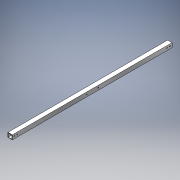
# Autodesk Inventor part: 上昇機構_角柱3
Saved by Autodesk Inventor 2019.4 (Build 234330000, 330)
## iProperties
Created: 2021-12-04
Part Number: 上昇機構_角柱3
Material: アルミニウム 6061
Document SubType Name: Modeling
Designer: 堀川皓史
Density: 2.7 g/cm^3
Appearance: アルミニウム - フラット
Mass: 119.894 g
Surface Area: 595.499 cm^2
Volume: 44.4052 cm^3
Author: 堀川皓史
Autodesk Inventor part; units mm, degrees
ref_plane "YZ Plane" through (0, 0, 0) normal (1, 0, 0) x (0, 1, 0)
ref_plane "XZ Plane" through (0, 0, 0) normal (0, 1, 0) x (-1, 0, 0)
ref_plane "XY Plane" through (0, 0, 0) normal (0, 0, 1) x (1, 0, 0)
sketch "スケッチ1" plane through (0, 0, 0) normal (0, 0, 1) x (1, 0, 0)
  line L0 (7.5, 7.5) -> (-7.5, 7.5)
  line L1 (-7.5, 7.5) -> (-7.5, -7.5)
  line L2 (-7.5, -7.5) -> (7.5, -7.5)
  line L3 (7.5, -7.5) -> (7.5, 7.5)
  line L4 (7.5, 7.5) -> (-7.5, -7.5) construction
  line L5 (-7.5, 7.5) -> (7.5, -7.5) construction
  line L6 (-6, 6) -> (6, 6)
  line L7 (6, 6) -> (6, -6)
  line L8 (6, -6) -> (-6, -6)
  line L9 (-6, -6) -> (-6, 6)
  point P0 (0, 0)
  dimension "d0" = 15
  dimension "d1" = 15
  dimension "d2" = 1.5
  constraints: 20 end point, 4 parallel, 2 midpoint, 2 perpendicular, 1 horizontal, 3 other
  measures "d0" distance of L2.end L1.end
  measures "d1" distance of L1.end L0.end
  measures "d2" distance between parallel lines of L0 L6
extrude "押し出し1" add sketch "スケッチ1" along normal blind 550
sketch "スケッチ2" plane through (7.5, -7.5, 0) normal (1, 0, 0) x (0, 0, -1)
  circle A0 centre (-7, 7.5) radius 1.6
  circle A1 centre (-17, 7.5) radius 1.6
  line L0 (0, 0) -> (0, 15) projected
  circle A2 centre (-533, 7.5) radius 1.6
  circle A3 centre (-543, 7.5) radius 1.6
  line L1 (-550, 0) -> (-550, 15) projected
  circle A4 centre (-254, 7.5) radius 1.6
  circle A5 centre (-294, 7.5) radius 1.6
  point P0 (0, 7.5)
  point P1 (0, 7.5)
  dimension "d5" = 3.2
  dimension "d6" = 3.2
  dimension "d7" = 7
  dimension "d8" = 10
  dimension "d9" = 3.2
  dimension "d10" = 3.2
  dimension "d11" = 10
  dimension "d12" = 7
  dimension "d13" = 3.2
  dimension "d14" = 3.2
  dimension "d15" = 40
  dimension "d19" = 237
  constraints: 6 centre point, 6 horizontal alignment, 1 midpoint
  measures "d5" diameter of A0
  measures "d6" diameter of A1
  measures "d7" distance of point (0, 7.5) A0.centre
  measures "d8" distance of A0.centre A1.centre
  measures "d9" diameter of A2
  measures "d10" diameter of A3
  measures "d11" distance of A2.centre A3.centre
  measures "d12" distance from line of L1 A3.centre
  measures "d13" diameter of A4
  measures "d14" diameter of A5
  measures "d15" distance of A4.centre A5.centre
  measures "d19" distance of A1.centre A4.centre
extrude "押し出し2" cut sketch "スケッチ2" against normal through all
